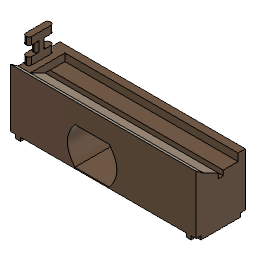
Projectile Base (Autodesk Fusion 360 design; units mm, degrees)
part number: 2026-05-27-21-07-16-421
Autodesk Fusion 360 part; units mm, degrees
sketch "Sketch12" plane through (0, 0, 0) normal (0, 1, 0) x (1, 0, 0)
  line L0 (0, 0) -> (66, 0)
  line L1 (66, 0) -> (66, -20)
  line L2 (66, -20) -> (0, -20)
  line L3 (0, -9) -> (0, -8)
  line L4 (0, 0) -> (0, -3)
  line L5 (0, -3) -> (66, -3)
  line L6 (0, -20) -> (0, -17)
  line L7 (0, -17) -> (66, -17)
  line L8 (0, -9) -> (66, -9)
  line L9 (0, -11) -> (66, -11)
  line L10 (0, -20) -> (0, -11)
  line L11 (0, -9) -> (0, 0)
  line L12 (0, -9) -> (0, -11)
  dimension "d95" = 1
  constraint horizontal L0
  constraint vertical L1
  constraint horizontal L2
  constraint vertical L10
  constraint coincident L0.start L4.start
  constraint coincident L4.end L11
  constraint coincident L1 L5.end
  constraint perpendicular L1 L5
  constraint coincident L6.end L10
  constraint coincident L1 L7.end
  constraint perpendicular L1 L7
  constraint coincident L1 L8.end
  constraint perpendicular L1 L8
  constraint coincident L1 L9.end
  constraint perpendicular L1 L9
  constraint collinear L10 L11
  measures "d95" distance of L3.start L3.end
extrude "Extrude29" add sketch "Sketch12" along normal blind 20 contours L1 L3 L5 L8 L11 | L1 L7 L9 L10 makes body 1 at (22, 6.6667, 3) makes body 2 at (22, 6.6667, 17)
extrude "Extrude30" add sketch "Sketch12" along normal blind 18 contours L1 L8 L9 L12 bodies 1 2
extrude "Extrude31" add sketch "Sketch12" along normal blind 23 contours L1 L2 L6 L7 L10 bodies 1
extrude "Extrude32" add sketch "Sketch12" along normal blind 23 contours L0 L1 L4 L5 L11 bodies 1
sketch "Sketch13" plane through (0, 0, 3) normal (0, 0, 1) x (1, 0, 0)
  line L0 (0, 20) -> (66, 20)
  line L1 (66, 20) -> (66, 23)
  line L2 (66, 23) -> (0, 23)
  line L3 (0, 23) -> (0, 20)
  line L4 (0, 23) -> (3.4404, 23)
  line L5 (3.4404, 23) -> (3.4404, 20)
  line L6 (3.4404, 20) -> (0, 20)
  line L7 (0, 20) -> (0, 23)
  constraint horizontal L4
  constraint vertical L5
  constraint horizontal L6
  constraint vertical L7
  constraint coincident L0 L5.end
  constraint coincident L2.end L3.start
extrude "Extrude33" add sketch "Sketch13" along normal blind 6 contours L0 L2 L3 L4 L5 L6 L7 bodies 1
sketch "Sketch14" plane through (0, 0, 17) normal (0, 0, -1) x (-1, 0, 0)
  line L0 (-66, 20) -> (0, 20)
  line L1 (0, 20) -> (0, 23)
  line L2 (0, 23) -> (-66, 23)
  line L3 (-66, 23) -> (-66, 20)
  line L4 (0, 23) -> (-3, 23)
  line L5 (-3, 23) -> (-3, 20)
  line L6 (-3, 20) -> (0, 20)
  line L7 (0, 20) -> (0, 23)
  constraint horizontal L4
  constraint vertical L5
  constraint horizontal L6
  constraint vertical L7
  constraint coincident L0 L5.end
  constraint coincident L1.end L2.start
extrude "Extrude34" add sketch "Sketch14" along normal blind 6 contours L0 L1 L2 L4 L5 L6 L7 bodies 1
extrude "Extrude35" add 1 faces at (66, 6, 10.3333) along direction (1, 0, 0) blind 10 on bodies 1 bodies 1
sketch "Sketch15" plane through (0, 0, 0) normal (0, 0, -1) x (-1, 0, 0)
  line L0 (-76, 0) -> (0, 0)
  line L1 (0, 0) -> (0, 23)
  line L2 (0, 23) -> (-76, 23)
  line L3 (-76, 23) -> (-76, 0)
  line L4 (-76, 0) -> (-38, 0)
  line L5 (-38, 0) -> (-38, 11.5)
  circle A0 centre (-38, 11.5) radius 1
  dimension "d110" = 11.5
  dimension "d111" = 2
  constraint coincident L0.start L3.end
  constraint midpoint L0 L4.end
  constraint perpendicular L2 L5
  constraint coincident L5.end A0.centre
  measures "d110" distance of L4.end L5.end
  measures "d111" diameter of A0
sketch "Sketch16" plane through (0, 23, 0) normal (0, 1, 0) x (-1, 0, 0)
  line L0 (0, 20) -> (-76, 20)
  line L1 (-76, 20) -> (-76, 17)
  line L2 (-76, 17) -> (-3, 17)
  line L3 (-3, 17) -> (-3, 11)
  line L4 (-3, 11) -> (0, 11)
  line L5 (0, 11) -> (0, 20)
  line L6 (0, 20) -> (0, 0)
  line L7 (0, 0) -> (-10, 0)
  line L8 (-10, 0) -> (-10, 20)
  line L9 (0, 20) -> (-10, 20)
  constraint coincident L0.start L5.end
  constraint coincident L6.end L7.start
  constraint perpendicular L5 L7
  constraint coincident L0 L8.end
  constraint perpendicular L0 L8
extrude "Extrude36" add sketch "Sketch16" against normal blind 3 contours L0 L2 L3 L4 L5 L6 L8 L9 | L2 L3 L4 L6 L7 L8 bodies 1
sketch "Sketch17" plane through (0, 23, 0) normal (0, 1, 0) x (-1, 0, 0)
  line L0 (-10, 17) -> (-10, 3)
  line L1 (-10, 3) -> (-76, 3)
  line L2 (-76, 3) -> (-76, 0)
  line L3 (-76, 0) -> (0, 0)
  line L4 (0, 0) -> (0, 20)
  line L5 (0, 20) -> (-76, 20)
  line L6 (-76, 20) -> (-76, 17)
  line L7 (-76, 17) -> (-10, 17)
  line L8 (0, 0) -> (0, 20)
  line L9 (0, 0) -> (0, 10)
  line L10 (-2.5, 5) -> (-2.5, 15)
  line L11 (-2.5, 5) -> (-7.5, 5)
  line L12 (-7.5, 5) -> (-7.5, 15)
  line L13 (-7.5, 15) -> (-2.5, 15)
  line L14 (-2.5, 15) -> (-2.5, 5)
  dimension "d114" = 10
  dimension "d117" = 10
  dimension "d118" = 5
  dimension "d119" = 10
  constraint coincident L3.end L4.start
  constraint coincident L4.end L5.start
  constraint perpendicular L5 L9
  constraint horizontal L11
  constraint vertical L12
  constraint horizontal L13
  constraint vertical L14
  measures "d114" distance of L3.end L9.end
  measures "d117" distance of L10.start L10.end
  measures "d118" distance of L10.start L11.end
  measures "d119" distance of L10.start L10.end
extrude "Extrude37" add sketch "Sketch17" along normal blind 10 contours L10 L11 L12 L13 L14 bodies 1
sketch "Sketch18" plane through (0, 0, 5) normal (0, 0, -1) x (-1, 0, 0)
  line L0 (-7.5, 23) -> (-2.5, 23)
  line L1 (-2.5, 23) -> (-2.5, 33)
  line L2 (-2.5, 33) -> (-7.5, 33)
  line L3 (-7.5, 33) -> (-7.5, 23)
  line L4 (-2.5, 33) -> (-2.5, 30)
  line L5 (-2.5, 30) -> (-7.5, 30)
  line L6 (-7.5, 30) -> (-7.5, 26)
  line L7 (-7.5, 26) -> (-2.5, 26)
  line L8 (-2.5, 26) -> (-2.5, 30)
  dimension "d122" = 4
  constraint coincident L1.end L2.start
  constraint coincident L1 L4.end
  constraint horizontal L5
  constraint vertical L6
  constraint horizontal L7
  constraint vertical L8
  measures "d122" distance of L4.end L7.end
extrude "Extrude38" cut sketch "Sketch18" against normal blind 3 contours L1 L3 L5 L6 L7 L8 bodies 1
sketch "Sketch19" plane through (0, 0, 15) normal (0, 0, 1) x (1, 0, 0)
  line L0 (2.5, 23) -> (7.5, 23)
  line L1 (7.5, 23) -> (7.5, 33)
  line L2 (7.5, 33) -> (2.5, 33)
  line L3 (2.5, 33) -> (2.5, 23)
  line L4 (7.5, 33) -> (7.5, 30)
  line L5 (7.5, 30) -> (2.5, 30)
  line L6 (2.5, 30) -> (2.5, 26)
  line L7 (2.5, 26) -> (7.5, 26)
  line L8 (7.5, 26) -> (7.5, 30)
  dimension "d125" = 3
  dimension "d126" = 4
  constraint coincident L1.end L2.start
  constraint perpendicular L2 L4
  constraint horizontal L5
  constraint vertical L6
  constraint horizontal L7
  constraint vertical L8
  measures "d125" distance of L1.end L4.end
  measures "d126" distance of L4.end L7.end
extrude "Extrude39" cut sketch "Sketch19" against normal blind 3 contours L1 L3 L5 L6 L7 L8 bodies 1
extrude "Extrude40" add 1 faces at (2.5, 24, 10.6667) along direction (-1, 0, 0) blind 2.5 on bodies 1 bodies 1
sketch "Sketch20" plane through (0, 0, 20) normal (0, 0, 1) x (1, 0, 0)
  line L0 (76, 23) -> (0, 23)
  line L1 (0, 23) -> (0, 0)
  line L2 (0, 0) -> (76, 0)
  line L3 (76, 0) -> (76, 23)
  circle A0 centre (38, 9.5) radius 1
  line L4 (38, 17) -> (45, 17)
  line L5 (38, 17) -> (31, 17)
  line L6 (38, 2) -> (45, 2)
  line L7 (38, 2) -> (31, 2)
  spline S0 degree 5 poles (31, 17) (30.7725, 16.7) (30.3372, 16.1) (29.744, 15.2) (29.0743, 14) (28.4528, 12.5) (28.0663, 11) (27.934, 9.5) (28.0663, 8) (28.4528, 6.5) (29.0743, 5) (29.744, 3.8) (30.3372, 2.9) (30.7725, 2.3) (31, 2) knots 0 0 0 0 0 0 0.1 0.2 0.3 0.4 0.5 0.6 0.7 0.8 0.9 1 1 1 1 1 1
  spline S1 degree 5 poles (45, 17) (45.2275, 16.7) (45.6628, 16.1) (46.256, 15.2) (46.9257, 14) (47.5472, 12.5) (47.9337, 11) (48.066, 9.5) (47.9337, 8) (47.5472, 6.5) (46.9257, 5) (46.256, 3.8) (45.6628, 2.9) (45.2275, 2.3) (45, 2) knots 0 0 0 0 0 0 0.1 0.2 0.3 0.4 0.5 0.6 0.7 0.8 0.9 1 1 1 1 1 1
  point P0 (48, 9.5)
  point P1 (28, 9.5)
  dimension "d138" = 2
  dimension "d139" = 10
  dimension "d140" = 10
  dimension "d141" = 7.5
  dimension "d142" = 7.5
  dimension "d143" = 7
  dimension "d144" = 7
  dimension "d145" = 7
  dimension "d146" = 7
  measures "d138" diameter of A0
  measures "d139" distance of A0.centre P0
  measures "d140" distance of A0.centre P1
  measures "d141" distance of A0.centre L4.start
  measures "d142" distance of A0.centre L6.start
  measures "d143" distance of L4.start L4.end
  measures "d144" distance of L4.start L5.end
  measures "d145" distance of L6.start L6.end
  measures "d146" distance of L6.start L7.end
extrude "Extrude41" cut sketch "Sketch20" against normal blind 19 contours L4 L5 L6 L7 S0 S1 bodies 1
extrude "Extrude42" cut 1 faces at (37.5121, 9.7267, 20) along direction (0, 0, -1) blind 45 on bodies 1 bodies 1
sketch "Sketch21" plane through (0, 0, 20) normal (0, 0, 1) x (1, 0, 0)
  line L0 (76, 23) -> (0, 23)
  line L1 (0, 23) -> (0, 0)
  line L2 (0, 0) -> (76, 0)
  line L3 (76, 0) -> (76, 23)
  spline S0 degree 5 poles (31, 2) (30.7725, 2.3) (30.3372, 2.9) (29.744, 3.8) (29.0743, 5) (28.4528, 6.5) (28.0663, 8) (27.934, 9.5) (28.0663, 11) (28.4528, 12.5) (29.0743, 14) (29.744, 15.2) (30.3372, 16.1) (30.7725, 16.7) (31, 17) knots -1 -1 -1 -1 -1 -1 -0.9 -0.8 -0.7 -0.6 -0.5 -0.4 -0.3 -0.2 -0.1 0 0 0 0 0 0
  line L4 (31, 17) -> (45, 17)
  spline S1 degree 5 poles (45, 17) (45.2275, 16.7) (45.6628, 16.1) (46.256, 15.2) (46.9257, 14) (47.5472, 12.5) (47.9337, 11) (48.066, 9.5) (47.9337, 8) (47.5472, 6.5) (46.9257, 5) (46.256, 3.8) (45.6628, 2.9) (45.2275, 2.3) (45, 2) knots 0 0 0 0 0 0 0.1 0.2 0.3 0.4 0.5 0.6 0.7 0.8 0.9 1 1 1 1 1 1
  line L5 (45, 2) -> (31, 2)
  line L6 (0, 23) -> (76, 23)
  line L7 (76, 23) -> (76, 21)
  line L8 (76, 21) -> (0, 21)
  line L9 (0, 21) -> (0, 23)
  constraint horizontal L6
  constraint vertical L7
  constraint horizontal L8
  constraint vertical L9
  constraint coincident L3 L7.end
  constraint coincident L0.end L1.start
extrude "Extrude43" add sketch "Sketch21" along normal blind 20 contours L0 L1 L3 L6 L7 L8 L9 bodies 1
sketch "Sketch22" plane through (0, 23, 0) normal (0, 1, 0) x (-1, 0, 0)
  line L0 (0, 5) -> (-7.5, 5)
  line L1 (-7.5, 5) -> (-7.5, 15)
  line L2 (-7.5, 15) -> (0, 15)
  line L3 (0, 15) -> (0, 40)
  line L4 (0, 40) -> (-76, 40)
  line L5 (-76, 40) -> (-76, 17)
  line L6 (-76, 17) -> (-10, 17)
  line L7 (-10, 17) -> (-10, 3)
  line L8 (-10, 3) -> (-76, 3)
  line L9 (-76, 3) -> (-76, 0)
  line L10 (-76, 0) -> (0, 0)
  line L11 (-76, 17) -> (0, 17)
  line L12 (0, 17) -> (0, 20)
  line L13 (0, 20) -> (-76, 20)
  line L14 (-76, 20) -> (-76, 17)
  line L15 (-76, 20) -> (0, 20)
  line L16 (0, 20) -> (0, 40)
  line L17 (0, 40) -> (-76, 40)
  line L18 (-76, 40) -> (-76, 20)
  line L19 (0, 0) -> (0, 5)
  constraint horizontal L11
  constraint vertical L12
  constraint horizontal L13
  constraint vertical L14
  constraint coincident L3 L12.end
  constraint coincident L5.end L6.start
  constraint horizontal L15
  constraint vertical L16
  constraint horizontal L17
  constraint vertical L18
  constraint coincident L3.end L4.start
extrude "Extrude44" cut 1 faces at (50.6667, 21, 26.6667) along direction (0, 1, 0) blind 10 on bodies 1 bodies 1
extrude "Extrude45" add sketch "Sketch22" along normal blind 20 separate body contours L3 L4 L5 L13 L15 L16 L17 L18 makes body 3
draft "Draft1" angle 15 neutral plane through (0, 0, 0) pull (0, 0, 1) 1 faces at (50.6667, 23, 33.3333) on bodies 3
move_body "Move1" bodies 3 to x (1, 0, 0) y (0, 1, 0) z (0, 0, 1) at (0, -5, 0)
move_body "Move2" bodies 3 to x (1, 0, 0) y (0, 1, 0) z (0, 0, 1) at (0, 0, -1)
move_body "Move3" bodies 3 to x (1, 0, 0) y (0, 1, 0) z (0, 0, 1) at (0, 0, 1)
sketch "Sketch23" plane through (0, 0, 20) normal (0, 0, -1) x (-1, 0, 0)
  line L0 (-76, 23.359) -> (0, 23.359)
  line L1 (0, 23.359) -> (0, 38)
  line L2 (0, 38) -> (-76, 38)
  line L3 (-76, 38) -> (-76, 23.359)
  line L4 (-75, 24) -> (-10, 24)
  line L5 (-10, 24) -> (-10, 26)
  line L6 (-10, 26) -> (-75, 26)
  line L7 (-75, 26) -> (-75, 24)
  constraint parallel L0 L4
  constraint perpendicular L4 L5
  constraint perpendicular L5 L6
  constraint perpendicular L4 L7
draft "Draft2" angle -15 neutral plane through (0, 0, 0) pull (0, 0, 1) 1 faces at (50.6667, 26.9316, 33.3333) on bodies 3
extrude "Extrude46" cut sketch "Sketch23" against normal blind 7 contours L4 L5 L6 L7 bodies 3
extrude "Extrude47" add 1 faces at (76, 6, 9.6667) along direction (1, 0, 0) blind 5 on bodies 1 bodies 1 3
extrude "Extrude48" cut 1 faces at (81, 6, 9.6667) along direction (-1, 0, 0) blind 1 on bodies 1 bodies 1
extrude "Extrude49" cut 2 faces at (0, 6, 10.3333) (0, 26.3333, 33.3333) along direction (1, 0, 0) blind 5 on bodies 1 bodies 1
extrude "Extrude50" add 1 faces at (52.3333, 38, 33.3333) along direction (0, 1, 0) blind 8 on bodies 1 bodies 1
sketch "Sketch24" plane through (5, 0, 0) normal (-1, 0, 0) x (0, 0, 1)
  line L0 (20, 0) -> (20, 18)
  line L1 (20, 18) -> (40, 18)
  line L2 (40, 18) -> (40, 46)
  line L3 (40, 46) -> (20, 46)
  line L4 (20, 46) -> (20, 23)
  line L5 (20, 23) -> (15, 23)
  line L6 (15, 23) -> (15, 26)
  line L7 (15, 26) -> (12, 26)
  line L8 (12, 26) -> (12, 30)
  line L9 (12, 30) -> (15, 30)
  line L10 (15, 30) -> (15, 33)
  line L11 (15, 33) -> (5, 33)
  line L12 (5, 33) -> (5, 30)
  line L13 (5, 30) -> (8, 30)
  line L14 (8, 30) -> (8, 26)
  line L15 (8, 26) -> (5, 26)
  line L16 (5, 26) -> (5, 23)
  line L17 (5, 23) -> (0, 23)
  line L18 (0, 23) -> (0, 0)
  line L19 (0, 0) -> (20, 0)
  line L20 (11, 20) -> (11, 18)
  line L21 (11, 18) -> (9, 18)
  line L22 (9, 18) -> (9, 20)
  line L23 (9, 20) -> (11, 20)
  line L24 (0, 0) -> (2, 0)
  line L25 (2, 0) -> (2, 1.5)
  line L26 (2, 1.5) -> (0, 1.5)
  line L27 (0, 1.5) -> (0, 0)
  line L28 (20, 0) -> (18, 0)
  line L29 (18, 0) -> (18, 1.5)
  line L30 (18, 1.5) -> (20, 1.5)
  line L31 (20, 1.5) -> (20, 0)
  dimension "d171" = 2
  dimension "d172" = 1.5
  dimension "d173" = 2
  dimension "d174" = 1.5
  constraint horizontal L24
  constraint vertical L25
  constraint horizontal L26
  constraint vertical L27
  constraint coincident L18.end L19.start
  constraint horizontal L28
  constraint vertical L29
  constraint horizontal L30
  constraint vertical L31
  constraint coincident L0.start L19.end
  measures "d171" distance of L18.end L24.end
  measures "d172" distance of L18.end L26.end
  measures "d173" distance of L0.start L28.end
  measures "d174" distance of L0.start L30.end
extrude "Extrude51" cut sketch "Sketch24" against normal blind 79 contours L0 L19 L28 L29 L30 L31 | L18 L19 L24 L25 L26 L27 bodies 1
sketch "Sketch25" plane through (0, 0, 2) normal (0, 0, -1) x (-1, 0, 0)
  line L0 (-80, 1.5) -> (-80, 0)
  line L1 (-80, 0) -> (-5, 0)
  line L2 (-5, 0) -> (-5, 1.5)
  line L3 (-5, 1.5) -> (-80, 1.5)
  line L4 (-80, 0) -> (-78, 0)
  line L5 (-78, 0) -> (-78, 1.5)
  line L6 (-78, 1.5) -> (-80, 1.5)
  line L7 (-80, 1.5) -> (-80, 0)
  line L8 (-78, 0) -> (-76, 0)
  line L9 (-76, 0) -> (-76, 1.5)
  line L10 (-76, 1.5) -> (-78, 1.5)
  line L11 (-78, 1.5) -> (-78, 0)
  line L12 (-5, 0) -> (-7, 0)
  line L13 (-7, 0) -> (-7, 1.5)
  line L14 (-7, 1.5) -> (-5, 1.5)
  line L15 (-5, 1.5) -> (-5, 0)
  line L16 (-7, 0) -> (-9, 0)
  line L17 (-9, 0) -> (-9, 1.5)
  line L18 (-9, 1.5) -> (-7, 1.5)
  line L19 (-7, 1.5) -> (-7, 0)
  dimension "d177" = 2
  dimension "d178" = 2
  dimension "d179" = 2
  dimension "d180" = 2
  constraint horizontal L4
  constraint vertical L5
  constraint horizontal L6
  constraint vertical L7
  constraint coincident L0.end L1.start
  constraint horizontal L8
  constraint vertical L9
  constraint horizontal L10
  constraint vertical L11
  constraint horizontal L12
  constraint vertical L13
  constraint horizontal L14
  constraint vertical L15
  constraint coincident L1.end L2.start
  constraint horizontal L16
  constraint vertical L17
  constraint horizontal L18
  constraint vertical L19
  measures "d177" distance of L0.end L4.end
  measures "d178" distance of L4.end L8.end
  measures "d179" distance of L1.end L12.end
  measures "d180" distance of L12.end L16.end
extrude "Extrude52" add sketch "Sketch25" along normal blind 2 contours L1 L3 L5 L8 L9 L10 L11 | L1 L3 L13 L16 L17 L18 L19 bodies 1
sketch "Sketch26" plane through (0, 0, 18) normal (0, 0, 1) x (1, 0, 0)
  line L0 (80, 0) -> (80, 1.5)
  line L1 (80, 1.5) -> (5, 1.5)
  line L2 (5, 1.5) -> (5, 0)
  line L3 (5, 0) -> (80, 0)
  line L4 (5, 0) -> (7, 0)
  line L5 (7, 0) -> (7, 1.5)
  line L6 (7, 1.5) -> (5, 1.5)
  line L7 (5, 1.5) -> (5, 0)
  line L8 (7, 0) -> (9, 0)
  line L9 (9, 0) -> (9, 1.5)
  line L10 (9, 1.5) -> (7, 1.5)
  line L11 (7, 1.5) -> (7, 0)
  line L12 (80, 0) -> (78, 0)
  line L13 (78, 0) -> (78, 1.5)
  line L14 (78, 1.5) -> (80, 1.5)
  line L15 (80, 1.5) -> (80, 0)
  line L16 (78, 0) -> (76, 0)
  line L17 (76, 0) -> (76, 1.5)
  line L18 (76, 1.5) -> (78, 1.5)
  line L19 (78, 1.5) -> (78, 0)
  dimension "d183" = 2
  dimension "d184" = 2
  dimension "d185" = 2
  dimension "d186" = 2
  constraint horizontal L4
  constraint vertical L5
  constraint horizontal L6
  constraint vertical L7
  constraint coincident L2.end L3.start
  constraint horizontal L8
  constraint vertical L9
  constraint horizontal L10
  constraint vertical L11
  constraint horizontal L12
  constraint vertical L13
  constraint horizontal L14
  constraint vertical L15
  constraint coincident L0.start L3.end
  constraint horizontal L16
  constraint vertical L17
  constraint horizontal L18
  constraint vertical L19
  measures "d183" distance of L2.end L4.end
  measures "d184" distance of L4.end L8.end
  measures "d185" distance of L0.start L12.end
  measures "d186" distance of L12.end L16.end
extrude "Extrude53" add sketch "Sketch26" along normal blind 2 contours L1 L3 L13 L16 L17 L18 L19 | L1 L3 L5 L8 L9 L10 L11 bodies 1
extrude "Extrude54" cut 1 faces at (52.3333, 46, 33.3333) along direction (0, -1, 0) blind 44 on bodies 1 bodies 1
fillet "Fillet5" radius 1 4 edges at (5, 31.5, 5) (7.5, 31.5, 5) (7.5, 31.5, 15) (5, 31.5, 15) on bodies 1
fillet "Fillet6" radius 1 4 edges at (5, 28, 8) (7.5, 28, 8) (7.5, 28, 12) (5, 28, 12) on bodies 1
fillet "Fillet7" radius 1 4 edges at (5, 24.5, 5) (7.5, 24.5, 5) (7.5, 24.5, 15) (5, 24.5, 15) on bodies 1
sketch "Sketch27" plane through (80, 0, 0) normal (1, 0, 0) x (0, 0, -1)
  line L0 (-2, 1.5) -> (0, 1.5)
  line L1 (0, 1.5) -> (0, 23)
  line L2 (0, 23) -> (-3, 23)
  line L3 (-3, 23) -> (-3, 20)
  line L4 (-3, 20) -> (-9, 20)
  line L5 (-9, 20) -> (-9, 18)
  line L6 (-9, 18) -> (-11, 18)
  line L7 (-11, 18) -> (-11, 20)
  line L8 (-11, 20) -> (-17, 20)
  line L9 (-17, 20) -> (-17, 23)
  line L10 (-17, 23) -> (-20, 23)
  line L11 (-20, 23) -> (-20, 1.5)
  line L12 (-20, 1.5) -> (-18, 1.5)
  line L13 (-18, 1.5) -> (-18, 0)
  line L14 (-18, 0) -> (-2, 0)
  line L15 (-2, 0) -> (-2, 1.5)
  line L16 (-11, 20) -> (-17, 23)
  constraint coincident L7.end L8.start
  constraint coincident L9.end L10.start
extrude "Extrude57" add sketch "Sketch27" against normal blind 70 contours L8 L9 L16 bodies 1
sketch "Sketch28" plane through (80, 0, 0) normal (1, 0, 0) x (0, 0, -1)
  line L0 (-2, 1.5) -> (0, 1.5)
  line L1 (0, 1.5) -> (0, 23)
  line L2 (0, 23) -> (-3, 23)
  line L3 (-3, 23) -> (-3, 20)
  line L4 (-3, 20) -> (-9, 20)
  line L5 (-9, 20) -> (-9, 18)
  line L6 (-9, 18) -> (-11, 18)
  line L7 (-11, 18) -> (-11, 20)
  line L8 (-11, 20) -> (-17, 23)
  line L9 (-17, 23) -> (-20, 23)
  line L10 (-20, 23) -> (-20, 1.5)
  line L11 (-20, 1.5) -> (-18, 1.5)
  line L12 (-18, 1.5) -> (-18, 0)
  line L13 (-18, 0) -> (-2, 0)
  line L14 (-2, 0) -> (-2, 1.5)
  line L15 (-20, 23) -> (-20, 25.13)
  line L16 (-20, 25.13) -> (-17, 23)
  dimension "d206" = 2.13
  constraint coincident L9.end L10.start
  constraint perpendicular L9 L15
  constraint coincident L8.end L9.start
  measures "d206" distance of L9.end L15.end
extrude "Extrude58" add sketch "Sketch28" against normal blind 75 contours L9 L15 L16 bodies 1
sketch "Sketch29" plane through (0, 0, 0) normal (0, 0, -1) x (-1, 0, 0)
  line L0 (-80, 1.5) -> (-78, 1.5)
  line L1 (-78, 1.5) -> (-78, 0)
  line L2 (-78, 0) -> (-76, 0)
  line L3 (-76, 0) -> (-76, 1.5)
  line L4 (-76, 1.5) -> (-9, 1.5)
  line L5 (-9, 1.5) -> (-9, 0)
  line L6 (-9, 0) -> (-7, 0)
  line L7 (-7, 0) -> (-7, 1.5)
  line L8 (-7, 1.5) -> (-5, 1.5)
  line L9 (-5, 1.5) -> (-5, 23)
  line L10 (-5, 23) -> (-80, 23)
  line L11 (-80, 23) -> (-80, 1.5)
  circle A0 centre (-38, 9.5) radius 1
  circle A1 centre (-38, 9.5) radius 2.975
extrude "Extrude59" add 1 faces at (38.0249, 14.8324, 1) along direction (0, 0, 1) blind 1 on bodies 1 bodies 1
extrude "Extrude60" cut sketch "Sketch29" against normal blind 2 contours A1 bodies 1
extrude "Extrude61" add 1 faces at (38.0741, 3.5111, 2) along direction (0, 0, 1) blind 2 on bodies 1 bodies 1
extrude "Extrude62" cut 1 faces at (38.0741, 3.5111, 4) along direction (0, 0, -1) blind 2 on bodies 1 bodies 1
equation "d110 = ( 2.3 / 2 ) * 1 cm"
equation "d141 = ( 1.5 / 2 ) * 1 cm"
equation "d142 = ( 1.5 / 2 ) * 1 cm"
equation "d143 = ( 1.4 / 2 ) * 1 cm"
equation "d144 = ( 1.4 / 2 ) * 1 cm"
equation "d145 = ( 1.4 / 2 ) * 1 cm"
equation "d146 = ( 1.4 / 2 ) * 1 cm"
